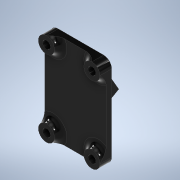
# Autodesk Inventor part: Case
Saved by Autodesk Inventor 2022 (Build 260153000, 153)
## iProperties
Created: 2021-03-01
Part Number: Case
Material: PET Plastic
Document SubType Name: Modeling
Designer: juanp
Density: 1.541 g/cm^3
Appearance: Polycarbonate - Clear
Author: juanp
Autodesk Inventor part; units mm, degrees
ref_plane "YZ Plane" through (0, 0, 0) normal (1, 0, 0) x (0, 1, 0)
ref_plane "XZ Plane" through (0, 0, 0) normal (0, 1, 0) x (-1, 0, 0)
sketch "Sketch1" plane through (0, 0, 0) normal (0, 0, 1) x (1, 0, 0)
  line L0 (2.2, 0) -> (14.7, 0)
  line L1 (16.9, 2.2) -> (16.9, 23.2)
  line L2 (14.7, 25.4) -> (2.2, 25.4)
  line L3 (0, 23.2) -> (0, 2.2)
  circle A0 centre (2.2, 2.2) radius 1.075
  circle A1 centre (14.7, 2.2) radius 1.075
  circle A2 centre (14.7, 23.2) radius 1.075
  circle A3 centre (2.2, 23.2) radius 1.075
  line L4 (2.2, 23.2) -> (14.7, 23.2) construction
  line L5 (14.7, 23.2) -> (14.7, 2.2) construction
  line L6 (14.7, 2.2) -> (2.2, 2.2) construction
  line L7 (2.2, 2.2) -> (2.2, 23.2) construction
  arc A4 (2.2, 25.4) -> (0, 23.2) centre (2.2, 23.2) ccw
  arc A5 (16.9, 23.2) -> (14.7, 25.4) centre (14.7, 23.2) ccw
  arc A6 (14.7, 0) -> (16.9, 2.2) centre (14.7, 2.2) ccw
  arc A7 (0, 2.2) -> (2.2, 0) centre (2.2, 2.2) ccw
  point P0 (0, 0)
  dimension "d2" = 2.15
  dimension "d3" = 2.2
  dimension "d4" = 2.2
  dimension "d5" = 2.2
  dimension "d6" = 2.2
  dimension "d7" = 12.5
  dimension "d8" = 21
  dimension "d9" = 2.2
  constraints: 16 end point, 8 centre point, 8 point on circle, 8 tangent, 6 equal radius, 4 coincident, 4 parallel, 2 horizontal, 2 perpendicular, 2 point on line
  measures "d2" diameter of A2
  measures "d3" distance from line of L3 A3.centre
  measures "d4" distance from line of L1 A2.centre
  measures "d5" distance from line of L0 A0.centre
  measures "d6" distance between parallel lines of L2 L4
  measures "d7" distance of L5.end L6.end
  measures "d8" distance between parallel lines of L6 L4
  measures "d9" radius of A4
extrude "Extrusion1" add sketch "Sketch1" along normal blind 1.5
sketch "Sketch2" plane through (0, 0, 1.5) normal (0, 0, 1) x (1, 0, 0)
  circle A0 centre (2.2, 2.2) radius 1.075 projected
  circle A1 centre (2.2, 23.2) radius 1.075 projected
  circle A2 centre (14.7, 23.2) radius 1.075 projected
  circle A3 centre (14.7, 2.2) radius 1.075 projected
  circle A4 centre (2.2, 23.2) radius 2.2
  circle A5 centre (14.7, 23.2) radius 2.2
  circle A6 centre (2.2, 2.2) radius 1.075 projected
  circle A7 centre (2.2, 2.2) radius 2.2
  circle A8 centre (14.7, 2.2) radius 1.075 projected
  circle A9 centre (14.7, 2.2) radius 2.2
  arc A10 (2.2, 25.4) -> (0, 23.2) centre (2.2, 23.2) ccw projected
  arc A11 (16.9, 23.2) -> (14.7, 25.4) centre (14.7, 23.2) ccw projected
  arc A12 (14.7, 0) -> (16.9, 2.2) centre (14.7, 2.2) ccw projected
  arc A13 (0, 2.2) -> (2.2, 0) centre (2.2, 2.2) ccw projected
  point P0 (0, 0)
  constraints: 4 centre point, 4 coincident, 4 concentric
extrude "Extrusion2" add sketch "Sketch2" along normal blind 1.734
fillet "Fillet1" radius 1.734 6 edges at (3.7556, 0.6444, 1.5) (2.2, 4.4, 1.5) (13.1444, 3.7556, 1.5) (13.1444, 21.6444, 1.5) (2.2, 21, 1.5) (3.7556, 24.7556, 1.5)
ref_plane "Work Plane3" through (14.7, 25.4, 0) normal (0, 0.5, -0.8660254) x (-1, 0, 0)
sketch "Sketch6" plane through (14.7, 25.4, 0) normal (0, 0.5, -0.8660254) x (-1, 0, 0)
  line L0 (0, 0) -> (12.5, 0) projected
  line L1 (10.0969, -16.5) -> (4.0969, -16.5)
  line L2 (4.0969, -16.5) -> (4.0969, 0)
  line L3 (4.0969, 0) -> (10.0969, 0)
  line L4 (10.0969, 0) -> (10.0969, -16.5)
  point P0 (14.7, -21.997)
  point P1 (6.25, 0)
  dimension "d30" = 16.5
  dimension "d64" = 2.1531
  dimension "d65" = 3.8469
  constraints: 8 end point, 2 parallel, 1 collinear, 1 horizontal, 1 midpoint, 1 perpendicular
  measures "d30" distance between parallel lines of L1 L0
  measures "d64" distance from line of point (6.25, 0) L2
  measures "d65" distance from line of L4 point (6.25, 0)
ref_plane "Work Plane4" through (4.6031, 11.1106, -8.25) normal (0, 0.8660254, 0.5) x (1, 0, 0)
sketch "Sketch7" plane through (4.6031, 11.1106, -8.25) normal (0, 0.8660254, 0.5) x (1, 0, 0)
  line L0 (0, 0) -> (6, 0) projected
  line L1 (0, 0) -> (6, 0)
  line L2 (6, 0) -> (6, -3.75)
  line L3 (6, -3.75) -> (0, -3.75)
  line L4 (0, -3.75) -> (0, 0)
  point P0 (-4.6031, -12.7)
  dimension "d33" = 3.75
  constraints: 8 end point, 2 parallel, 1 horizontal, 1 perpendicular
  measures "d33" distance between parallel lines of L0 L3
extrude "Extrusion6" add sketch "Sketch7" along normal up to surface surface through (8.45, 12.7, 0) normal (0, 0, 1)
fillet "Fillet3" radius 4 1 edges at (7.6031, 17.9, 0)
sketch "Sketch19" plane through (4.6031, 5.3632, 0) normal (-1, 0, 0) x (0, 0, 1)
  line L0 (-8.25, 5.7474) -> (-5.0024, 3.8724) projected
  line L1 (-5.6519, 4.2474) -> (-3.1519, 8.5775) construction
  circle A0 centre (-3.1519, 8.5775) radius 1.1
  line L2 (-8.25, 5.7474) -> (0, 20.0368) projected
  point P0 (0, -5.3632)
  dimension "d67" = 2.2
  dimension "d68" = 5
  dimension "d71" = 3
  constraints: 2 end point, 1 centre point, 1 coincident, 1 perpendicular, 1 point on line
  measures "d67" diameter of A0
  measures "d68" distance of L1.start L1.end
  measures "d71" distance between parallel lines of L2 L1
extrude "Extrusion15" cut sketch "Sketch19" against normal through all
sketch "Sketch22" plane through (4.6031, 5.3632, 0) normal (-1, 0, 0) x (0, 0, 1)
  circle A0 centre (-3.1519, 8.5775) radius 1.1 projected
  line L0 (-1.9886, 10.5925) -> (-0.8252, 8.5775)
  line L1 (-0.8252, 8.5775) -> (-1.9886, 6.5625)
  line L2 (-1.9886, 6.5625) -> (-4.3153, 6.5625)
  line L3 (-4.3153, 6.5625) -> (-5.4786, 8.5775)
  line L4 (-5.4786, 8.5775) -> (-4.3153, 10.5925)
  line L5 (-4.3153, 10.5925) -> (-1.9886, 10.5925)
  line L6 (-8.25, 5.7474) -> (0, 20.0368) projected
  point P0 (0, -5.3632)
  dimension "d72" = 4.03
  constraints: 12 end point, 1 coincident, 1 parallel, 13 other
  measures "d72" distance between parallel lines of L4 L1
extrude "Extrusion16" cut sketch "Sketch22" against normal blind 1.5
body "Solid1"
